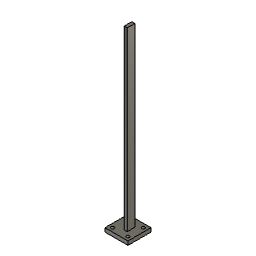
Sensor_mount_1 (Autodesk Fusion 360 design; units mm, degrees)
part number: 2025-07-07-15-14-59-097
Autodesk Fusion 360 part; units mm, degrees
sketch "Sketch1" plane through (0, 0, 0) normal (0, 0, 1) x (1, 0, 0)
  line L0 (0, 0) -> (30, 0)
  line L1 (30, 0) -> (30, 30)
  line L2 (30, 30) -> (0, 30)
  line L3 (0, 30) -> (0, 0)
  circle A0 centre (5, 25) radius 2
  circle A1 centre (25, 25) radius 2
  circle A2 centre (25, 5) radius 2
  circle A3 centre (5, 5) radius 2
  dimension "d1" = 30
  dimension "d2" = 30
  dimension "d3" = 4
  dimension "d4" = 5
  dimension "d5" = 5
  dimension "d6" = 4
  dimension "d7" = 4
  dimension "d8" = 4
  dimension "d9" = 20
  dimension "d10" = 20
  dimension "d11" = 20
  dimension "d12" = 20
  dimension "d13" = 5
  dimension "d14" = 5
  constraint horizontal L0
  constraint vertical L1
  constraint horizontal L2
  constraint vertical L3
  constraint coincident L0.start L3.end
  measures "d1" distance of L0.start L2.end
  measures "d2" distance of L0.start L0.end
  measures "d3" diameter of A0
  measures "d4" distance of L2 A0.centre
  measures "d5" distance of L3 A0.centre
  measures "d6" diameter of A1
  measures "d7" diameter of A2
  measures "d8" diameter of A3
  measures "d9" distance of A0.centre A3.centre
  measures "d10" distance of A2.centre A3.centre
  measures "d11" distance of A1.centre A2.centre
  measures "d12" distance of A0.centre A1.centre
  measures "d13" distance of L2 A1.centre
  measures "d14" distance of L0 A2.centre
extrude "Extrude1" add sketch "Sketch1" along normal blind 5
sketch "Sketch2" plane through (0, 0, 5) normal (0, 0, 1) x (-1, 0, 0)
  circle A0 centre (-5, -5) radius 2
  circle A1 centre (-25, -5) radius 2
  circle A2 centre (-5, -25) radius 2
  circle A3 centre (-25, -25) radius 2
  line L0 (0, -30) -> (0, 0)
  line L1 (0, 0) -> (-30, 0)
  line L2 (-30, 0) -> (-30, -30)
  line L3 (-30, -30) -> (0, -30)
  line L4 (-15, -20) -> (-19, -20)
  line L5 (-19, -20) -> (-19, -10)
  line L6 (-19, -10) -> (-15, -10)
  line L7 (-15, -10) -> (-15, -20)
  dimension "d17" = 4
  dimension "d18" = 10
  dimension "d19" = 15
  dimension "d20" = 10
  constraint horizontal L4
  constraint vertical L5
  constraint horizontal L6
  constraint vertical L7
  measures "d17" distance of L5.end L6.end
  measures "d18" distance of L4.start L6.end
  measures "d19" distance of L0 L7
  measures "d20" distance of L1 L6
extrude "Extrude3" add sketch "Sketch2" along normal blind 230 contours L4 L5 L6 L7
